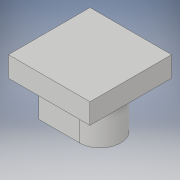
# Autodesk Inventor part: 6
Saved by Autodesk Inventor 2019 (Build 230136000, 136)
## iProperties
Created: 2018-08-10
Part Number: 6
Material: Generic
Document SubType Name: Modeling
Designer: Ge Shi
Density: 1 g/cm^3
Appearance: Default
Author: Ge Shi
Autodesk Inventor part; units mm, degrees
ref_plane "YZ Plane" through (0, 0, 0) normal (1, 0, 0) x (0, 1, 0)
ref_plane "XZ Plane" through (0, 0, 0) normal (0, 1, 0) x (-1, 0, 0)
ref_plane "XY Plane" through (0, 0, 0) normal (0, 0, 1) x (1, 0, 0)
sketch "Sketch1" plane through (0, 0, 0) normal (0, 1, 0) x (-1, 0, 0)
  line L0 (-10, -10) -> (10, -10)
  line L1 (10, -10) -> (10, 10)
  line L2 (10, 10) -> (-10, 10)
  line L3 (-10, 10) -> (-10, -10)
  line L4 (-10, -10) -> (10, 10) construction
  line L5 (10, -10) -> (-10, 10) construction
  circle A0 centre (-2.5, 0) radius 2.5
  arc A1 (-2.5, 5) -> (1.8301, 2.5) centre (-2.5, 0) ccw
  line L6 (-2.5, 5) -> (7.5, 5)
  line L7 (7.5, 5) -> (7.5, 2.5)
  line L8 (7.5, 2.5) -> (1.8301, 2.5)
  line L9 (-7.5, 0) -> (-7.5, -4.6851) construction
  line L10 (14, 0) -> (-14, 0) projected
  point P0 (0, 0)
  dimension "d0" = 20
  dimension "d1" = 20
  dimension "d2" = 2.5
  dimension "d3" = 2.5
  dimension "d4" = 2.5
  dimension "d5" = 2.5
  dimension "d6" = 5
  constraints: 20 end point, 3 perpendicular, 3 point on circle, 2 centre point, 2 horizontal, 2 midpoint, 2 parallel, 2 tangent, 1 coincident, 1 point on line, 1 vertical
  measures "d0" distance of L2.end L1.end
  measures "d1" distance of L0.end L1.end
  measures "d2" distance between parallel lines of L3 L9
  measures "d3" distance between parallel lines of L1 L7
  measures "d4" distance of L6.end L7.end
  measures "d5" radial gap between concentric circles of A0 A1
  measures "d6" radius of A1
extrude "Extrusion1" add sketch "Sketch1" against normal blind 10 contours L10 A0 A1 | A1 L6 L7 L8 L10 A0
extrude "Extrusion2" add sketch "Sketch1" along normal blind 5
body "Solid1"
